Autodesk Fusion 360 part; units mm, degrees
(part 2 of 2)
sketch "Sketch4" plane through (0, 0, 6.35) normal (0, 0, 1) x (-1, 0, 0)
  circle A0 centre (2.4092, -3.6756) radius 2.1488
  arc A1 (-0.9894, -8.6855) -> (-1.1636, -11.2308) centre (2.9194, -10.2316) ccw
  arc A2 (-1.1636, -11.2308) -> (-0.826, -11.3814) centre (2.4092, -3.6756) ccw
  arc A3 (-0.826, -11.3814) -> (0.9516, -9.5514) centre (-2.8101, -7.6757) ccw
  spline S0 degree 5 poles (0.9516, -9.5514) (0.9679, -9.5486) (1.0003, -9.5432) (1.0488, -9.5361) (1.1133, -9.5282) (1.1934, -9.5212) (1.273, -9.5171) (1.3428, -9.5162) (1.3964, -9.5173) (1.4342, -9.5189) (1.4562, -9.5202) (1.4625, -9.5206) knots 0 0 0 0 0 0 0.066667 0.133333 0.2 0.266667 0.333333 0.4 0.426673 0.426673 0.426673 0.426673 0.426673 0.426673
  spline S1 degree 5 poles (1.4625, -9.5206) (1.472, -9.5212) (1.4971, -9.5229) (1.5284, -9.5254) (1.5597, -9.5286) (1.591, -9.5324) (1.6129, -9.5353) (1.6191, -9.5361) knots 0.426673 0.426673 0.426673 0.426673 0.426673 0.426673 0.466667 0.533333 0.559717 0.559717 0.559717 0.559717 0.559717 0.559717
  spline S2 degree 5 poles (1.6191, -9.5361) (1.6253, -9.537) (1.6472, -9.54) (1.6783, -9.5446) (1.7094, -9.5498) (1.7402, -9.5556) (1.7649, -9.5607) (1.7742, -9.5626) knots -0.559717 -0.559717 -0.559717 -0.559717 -0.559717 -0.559717 -0.533333 -0.466667 -0.426673 -0.426673 -0.426673 -0.426673 -0.426673 -0.426673
  spline S3 degree 5 poles (1.7742, -9.5626) (1.7804, -9.5639) (1.8019, -9.5685) (1.8388, -9.5769) (1.8908, -9.5901) (1.9578, -9.6094) (2.0336, -9.6344) (2.109, -9.6624) (2.169, -9.6871) (2.2139, -9.7068) (2.2438, -9.7206) (2.2587, -9.7276) knots -0.426673 -0.426673 -0.426673 -0.426673 -0.426673 -0.426673 -0.4 -0.333333 -0.266667 -0.2 -0.133333 -0.066667 0 0 0 0 0 0
  arc A4 (2.2587, -9.7276) -> (3.4882, -11.963) centre (6.3829, -8.915) ccw
  arc A5 (3.4882, -11.963) -> (3.8537, -11.9072) centre (2.4092, -3.6756) ccw
  arc A6 (3.8537, -11.9072) -> (4.3597, -9.4066) centre (0.181, -9.8625) ccw
  spline S4 degree 5 poles (4.3597, -9.4066) (4.3718, -9.3955) (4.3962, -9.3734) (4.4332, -9.3412) (4.4831, -9.2997) (4.5467, -9.2505) (4.6115, -9.204) (4.6697, -9.1656) (4.7154, -9.1375) (4.7481, -9.1184) (4.7673, -9.1076) (4.7728, -9.1045) knots 0 0 0 0 0 0 0.066667 0.133333 0.2 0.266667 0.333333 0.4 0.426673 0.426673 0.426673 0.426673 0.426673 0.426673
  spline S5 degree 5 poles (4.7728, -9.1045) (4.7811, -9.0999) (4.8031, -9.0877) (4.8309, -9.073) (4.8589, -9.0587) (4.8873, -9.045) (4.9073, -9.0356) (4.9129, -9.0329) knots 0.426673 0.426673 0.426673 0.426673 0.426673 0.426673 0.466667 0.533333 0.559717 0.559717 0.559717 0.559717 0.559717 0.559717
  spline S6 degree 5 poles (4.9129, -9.0329) (4.9186, -9.0303) (4.9386, -9.021) (4.9674, -9.008) (4.9963, -8.9957) (5.0254, -8.9838) (5.0489, -8.9747) (5.0577, -8.9714) knots -0.559717 -0.559717 -0.559717 -0.559717 -0.559717 -0.559717 -0.533333 -0.466667 -0.426673 -0.426673 -0.426673 -0.426673 -0.426673 -0.426673
  spline S7 degree 5 poles (5.0577, -8.9714) (5.0636, -8.9691) (5.0843, -8.9613) (5.1198, -8.9485) (5.1707, -8.9314) (5.2375, -8.9114) (5.3148, -8.8915) (5.3933, -8.8743) (5.4572, -8.8626) (5.5056, -8.855) (5.5382, -8.8504) (5.5545, -8.8482) knots -0.426673 -0.426673 -0.426673 -0.426673 -0.426673 -0.426673 -0.4 -0.333333 -0.266667 -0.2 -0.133333 -0.066667 0 0 0 0 0 0
  arc A7 (5.5545, -8.8482) -> (7.7974, -10.064) centre (8.5847, -5.9349) ccw
  arc A8 (7.7974, -10.064) -> (8.0747, -9.8195) centre (2.4092, -3.6756) ccw
  arc A9 (8.0747, -9.8195) -> (7.1484, -7.4423) centre (3.8796, -10.085) ccw
  spline S8 degree 5 poles (7.1484, -7.4423) (7.1526, -7.4263) (7.1613, -7.3946) (7.1749, -7.3475) (7.1945, -7.2856) (7.2214, -7.2098) (7.2508, -7.1357) (7.2789, -7.0719) (7.3022, -7.0235) (7.3194, -6.9899) (7.3297, -6.9704) (7.3327, -6.9648) knots 0 0 0 0 0 0 0.066667 0.133333 0.2 0.266667 0.333333 0.4 0.426673 0.426673 0.426673 0.426673 0.426673 0.426673
  spline S9 degree 5 poles (7.3327, -6.9648) (7.3371, -6.9564) (7.3491, -6.9343) (7.3645, -6.9069) (7.3804, -6.8797) (7.3968, -6.8528) (7.4085, -6.8341) (7.4119, -6.8288) knots 0.426673 0.426673 0.426673 0.426673 0.426673 0.426673 0.466667 0.533333 0.559717 0.559717 0.559717 0.559717 0.559717 0.559717
  spline S10 degree 5 poles (7.4119, -6.8288) (7.4152, -6.8235) (7.427, -6.8049) (7.4442, -6.7785) (7.4618, -6.7524) (7.4799, -6.7267) (7.4948, -6.7063) (7.5004, -6.6987) knots -0.559717 -0.559717 -0.559717 -0.559717 -0.559717 -0.559717 -0.533333 -0.466667 -0.426673 -0.426673 -0.426673 -0.426673 -0.426673 -0.426673
  spline S11 degree 5 poles (7.5004, -6.6987) (7.5041, -6.6937) (7.5173, -6.676) (7.5402, -6.6459) (7.5738, -6.604) (7.6192, -6.5511) (7.6735, -6.4926) (7.7302, -6.4357) (7.7776, -6.3913) (7.8142, -6.3587) (7.8391, -6.3372) (7.8517, -6.3266) knots -0.426673 -0.426673 -0.426673 -0.426673 -0.426673 -0.426673 -0.4 -0.333333 -0.266667 -0.2 -0.133333 -0.066667 0 0 0 0 0 0
  arc A10 (7.8517, -6.3266) -> (10.3959, -6.1368) centre (8.8258, -2.2375) ccw
  arc A11 (10.3959, -6.1368) -> (10.4969, -5.7811) centre (2.4092, -3.6756) ccw
  arc A12 (10.4969, -5.7811) -> (8.4325, -4.2821) centre (7.1113, -8.2725) ccw
  spline S12 degree 5 poles (8.4325, -4.2821) (8.4274, -4.2664) (8.4175, -4.2351) (8.4035, -4.188) (8.3866, -4.1254) (8.3682, -4.0471) (8.3529, -3.9688) (8.342, -3.9) (8.3355, -3.8467) (8.3318, -3.809) (8.3299, -3.7871) (8.3294, -3.7808) knots 0 0 0 0 0 0 0.066667 0.133333 0.2 0.266667 0.333333 0.4 0.426673 0.426673 0.426673 0.426673 0.426673 0.426673
  spline S13 degree 5 poles (8.3294, -3.7808) (8.3286, -3.7714) (8.3267, -3.7462) (8.3248, -3.7149) (8.3235, -3.6834) (8.3227, -3.6519) (8.3225, -3.6298) (8.3225, -3.6236) knots 0.426673 0.426673 0.426673 0.426673 0.426673 0.426673 0.466667 0.533333 0.559717 0.559717 0.559717 0.559717 0.559717 0.559717
  spline S14 degree 5 poles (8.3225, -3.6236) (8.3224, -3.6173) (8.3222, -3.5953) (8.3224, -3.5637) (8.3232, -3.5323) (8.3245, -3.5009) (8.326, -3.4757) (8.3266, -3.4663) knots -0.559717 -0.559717 -0.559717 -0.559717 -0.559717 -0.559717 -0.533333 -0.466667 -0.426673 -0.426673 -0.426673 -0.426673 -0.426673 -0.426673
  spline S15 degree 5 poles (8.3266, -3.4663) (8.327, -3.46) (8.3285, -3.438) (8.3316, -3.4003) (8.3372, -3.3469) (8.3468, -3.2779) (8.3608, -3.1993) (8.3777, -3.1207) (8.3936, -3.0578) (8.4068, -3.0105) (8.4161, -2.979) (8.4209, -2.9633) knots -0.426673 -0.426673 -0.426673 -0.426673 -0.426673 -0.426673 -0.4 -0.333333 -0.266667 -0.2 -0.133333 -0.066667 0 0 0 0 0 0
  arc A13 (8.4209, -2.9633) -> (10.4586, -1.4281) centre (7.0297, 1.0033) ccw
  arc A14 (10.4586, -1.4281) -> (10.3514, -1.0743) centre (2.4092, -3.6756) ccw
  arc A15 (10.3514, -1.0743) -> (7.8042, -0.9293) centre (8.8501, -5.0006) ccw
  spline S16 degree 5 poles (7.8042, -0.9293) (7.7915, -0.9189) (7.7662, -0.8979) (7.729, -0.8659) (7.6808, -0.8224) (7.6231, -0.7664) (7.5678, -0.7089) (7.5215, -0.6568) (7.4872, -0.6155) (7.4637, -0.5859) (7.4502, -0.5684) (7.4464, -0.5634) knots 0 0 0 0 0 0 0.066667 0.133333 0.2 0.266667 0.333333 0.4 0.426673 0.426673 0.426673 0.426673 0.426673 0.426673
  spline S17 degree 5 poles (7.4464, -0.5634) (7.4407, -0.5559) (7.4255, -0.5358) (7.4069, -0.5104) (7.3888, -0.4847) (7.3712, -0.4586) (7.359, -0.4401) (7.3556, -0.4349) knots 0.426673 0.426673 0.426673 0.426673 0.426673 0.426673 0.466667 0.533333 0.559717 0.559717 0.559717 0.559717 0.559717 0.559717
  spline S18 degree 5 poles (7.3556, -0.4349) (7.3522, -0.4296) (7.3401, -0.4112) (7.3232, -0.3846) (7.3069, -0.3577) (7.291, -0.3305) (7.2786, -0.3086) (7.2741, -0.3003) knots -0.559717 -0.559717 -0.559717 -0.559717 -0.559717 -0.559717 -0.533333 -0.466667 -0.426673 -0.426673 -0.426673 -0.426673 -0.426673 -0.426673
  spline S19 degree 5 poles (7.2741, -0.3003) (7.271, -0.2948) (7.2604, -0.2755) (7.2426, -0.2421) (7.2184, -0.1942) (7.1892, -0.1309) (7.1585, -0.0573) (7.1302, 0.018) (7.1096, 0.0796) (7.0951, 0.1264) (7.0859, 0.158) (7.0814, 0.1739) knots -0.426673 -0.426673 -0.426673 -0.426673 -0.426673 -0.426673 -0.4 -0.333333 -0.266667 -0.2 -0.133333 -0.066667 0 0 0 0 0 0
  arc A16 (7.0814, 0.1739) -> (7.9657, 2.567) centre (3.7666, 2.7586) ccw
  arc A17 (7.9657, 2.567) -> (7.6842, 2.8066) centre (2.4092, -3.6756) ccw
  arc A18 (7.6842, 2.8066) -> (5.463, 1.5515) centre (8.544, -1.308) ccw
  spline S20 degree 5 poles (5.463, 1.5515) (5.4466, 1.5534) (5.414, 1.5574) (5.3654, 1.5642) (5.3014, 1.5748) (5.2226, 1.5906) (5.145, 1.6092) (5.0778, 1.6279) (5.0267, 1.6441) (4.9909, 1.6563) (4.9701, 1.6638) (4.9642, 1.6659) knots 0 0 0 0 0 0 0.066667 0.133333 0.2 0.266667 0.333333 0.4 0.426673 0.426673 0.426673 0.426673 0.426673 0.426673
  spline S21 degree 5 poles (4.9642, 1.6659) (4.9553, 1.6691) (4.9316, 1.6778) (4.9023, 1.6891) (4.8732, 1.701) (4.8442, 1.7134) (4.824, 1.7224) (4.8183, 1.7249) knots 0.426673 0.426673 0.426673 0.426673 0.426673 0.426673 0.466667 0.533333 0.559717 0.559717 0.559717 0.559717 0.559717 0.559717
  spline S22 degree 5 poles (4.8183, 1.7249) (4.8126, 1.7275) (4.7924, 1.7365) (4.7639, 1.7498) (4.7356, 1.7635) (4.7076, 1.7778) (4.6853, 1.7896) (4.677, 1.794) knots -0.559717 -0.559717 -0.559717 -0.559717 -0.559717 -0.559717 -0.533333 -0.466667 -0.426673 -0.426673 -0.426673 -0.426673 -0.426673 -0.426673
  spline S23 degree 5 poles (4.677, 1.794) (4.6714, 1.797) (4.652, 1.8075) (4.619, 1.826) (4.5728, 1.8533) (4.5139, 1.8907) (4.4483, 1.936) (4.3839, 1.9841) (4.3332, 2.0247) (4.2957, 2.0563) (4.2709, 2.0779) (4.2586, 2.0888) knots -0.426673 -0.426673 -0.426673 -0.426673 -0.426673 -0.426673 -0.4 -0.333333 -0.266667 -0.2 -0.133333 -0.066667 0 0 0 0 0 0
  arc A19 (4.2586, 2.0888) -> (3.7086, 4.5801) centre (0.0725, 2.4711) ccw
  arc A20 (3.7086, 4.5801) -> (3.3423, 4.6295) centre (2.4092, -3.6756) ccw
  arc A21 (3.3423, 4.6295) -> (2.1522, 2.3728) centre (6.2901, 1.6329) ccw
  spline S24 degree 5 poles (2.1522, 2.3728) (2.1374, 2.3655) (2.1078, 2.3512) (2.0633, 2.3307) (2.0037, 2.305) (1.9288, 2.2757) (1.8535, 2.2493) (1.7869, 2.2288) (1.7351, 2.2148) (1.6983, 2.2057) (1.6769, 2.2007) (1.6707, 2.1993) knots 0 0 0 0 0 0 0.066667 0.133333 0.2 0.266667 0.333333 0.4 0.426673 0.426673 0.426673 0.426673 0.426673 0.426673
  spline S25 degree 5 poles (1.6707, 2.1993) (1.6615, 2.1972) (1.6369, 2.1917) (1.6061, 2.1854) (1.5752, 2.1796) (1.5441, 2.1744) (1.5223, 2.171) (1.5161, 2.1701) knots 0.426673 0.426673 0.426673 0.426673 0.426673 0.426673 0.466667 0.533333 0.559717 0.559717 0.559717 0.559717 0.559717 0.559717
  spline S26 degree 5 poles (1.5161, 2.1701) (1.5099, 2.1691) (1.4881, 2.1659) (1.4569, 2.1616) (1.4256, 2.1578) (1.3944, 2.1547) (1.3693, 2.1526) (1.3598, 2.1518) knots -0.559717 -0.559717 -0.559717 -0.559717 -0.559717 -0.559717 -0.533333 -0.466667 -0.426673 -0.426673 -0.426673 -0.426673 -0.426673 -0.426673
  spline S27 degree 5 poles (1.3598, 2.1518) (1.3536, 2.1513) (1.3316, 2.1497) (1.2938, 2.1473) (1.2402, 2.1453) (1.1704, 2.145) (1.0907, 2.1476) (1.0105, 2.1532) (0.9459, 2.16) (0.8973, 2.1663) (0.8648, 2.1711) (0.8485, 2.1736) knots -0.426673 -0.426673 -0.426673 -0.426673 -0.426673 -0.426673 -0.4 -0.333333 -0.266667 -0.2 -0.133333 -0.066667 0 0 0 0 0 0
  arc A22 (0.8485, 2.1736) -> (-0.961, 3.9721) centre (-2.8797, 0.232) ccw
  arc A23 (-0.961, 3.9721) -> (-1.2959, 3.8155) centre (2.4092, -3.6756) ccw
  arc A24 (-1.2959, 3.8155) -> (-1.077, 1.2737) centre (2.804, 2.8884) ccw
  spline S28 degree 5 poles (-1.077, 1.2737) (-1.0855, 1.2596) (-1.1027, 1.2316) (-1.1291, 1.1902) (-1.1653, 1.1364) (-1.2125, 1.0712) (-1.2615, 1.0084) (-1.3065, 0.9551) (-1.3425, 0.9152) (-1.3685, 0.8878) (-1.3839, 0.872) (-1.3883, 0.8675) knots 0 0 0 0 0 0 0.066667 0.133333 0.2 0.266667 0.333333 0.4 0.426673 0.426673 0.426673 0.426673 0.426673 0.426673
  spline S29 degree 5 poles (-1.3883, 0.8675) (-1.3949, 0.8607) (-1.4126, 0.8428) (-1.4351, 0.8208) (-1.458, 0.7993) (-1.4813, 0.7781) (-1.4979, 0.7634) (-1.5026, 0.7593) knots 0.426673 0.426673 0.426673 0.426673 0.426673 0.426673 0.466667 0.533333 0.559717 0.559717 0.559717 0.559717 0.559717 0.559717
  spline S30 degree 5 poles (-1.5026, 0.7593) (-1.5072, 0.7552) (-1.5238, 0.7406) (-1.5478, 0.7201) (-1.572, 0.7001) (-1.5966, 0.6805) (-1.6166, 0.6651) (-1.6241, 0.6594) knots -0.559717 -0.559717 -0.559717 -0.559717 -0.559717 -0.559717 -0.533333 -0.466667 -0.426673 -0.426673 -0.426673 -0.426673 -0.426673 -0.426673
  spline S31 degree 5 poles (-1.6241, 0.6594) (-1.6291, 0.6556) (-1.6468, 0.6423) (-1.6773, 0.62) (-1.7213, 0.5893) (-1.7798, 0.5513) (-1.8483, 0.5104) (-1.9188, 0.4718) (-1.9767, 0.4425) (-2.0211, 0.4216) (-2.051, 0.408) (-2.0661, 0.4013) knots -0.426673 -0.426673 -0.426673 -0.426673 -0.426673 -0.426673 -0.4 -0.333333 -0.266667 -0.2 -0.133333 -0.066667 0 0 0 0 0 0
  arc A25 (-2.0661, 0.4013) -> (-4.5607, 0.936) centre (-4.1528, -3.2477) ccw
  arc A26 (-4.5607, 0.936) -> (-4.7578, 0.6232) centre (2.4092, -3.6756) ccw
  arc A27 (-4.7578, 0.6232) -> (-3.1994, -1.3967) centre (-0.8075, 2.0598) ccw
  spline S32 degree 5 poles (-3.1994, -1.3967) (-3.1989, -1.4132) (-3.1982, -1.4461) (-3.1981, -1.4951) (-3.1994, -1.56) (-3.2039, -1.6403) (-3.2112, -1.7197) (-3.2202, -1.7889) (-3.2289, -1.8418) (-3.2359, -1.879) (-3.2403, -1.9006) (-3.2416, -1.9068) knots 0 0 0 0 0 0 0.066667 0.133333 0.2 0.266667 0.333333 0.4 0.426673 0.426673 0.426673 0.426673 0.426673 0.426673
  spline S33 degree 5 poles (-3.2416, -1.9068) (-3.2435, -1.916) (-3.2488, -1.9407) (-3.2558, -1.9713) (-3.2634, -2.0019) (-3.2716, -2.0323) (-3.2776, -2.0535) (-3.2793, -2.0596) knots 0.426673 0.426673 0.426673 0.426673 0.426673 0.426673 0.466667 0.533333 0.559717 0.559717 0.559717 0.559717 0.559717 0.559717
  spline S34 degree 5 poles (-3.2793, -2.0596) (-3.281, -2.0656) (-3.2871, -2.0868) (-3.2961, -2.117) (-3.3057, -2.1469) (-3.3158, -2.1767) (-3.3243, -2.2004) (-3.3276, -2.2093) knots -0.559717 -0.559717 -0.559717 -0.559717 -0.559717 -0.559717 -0.533333 -0.466667 -0.426673 -0.426673 -0.426673 -0.426673 -0.426673 -0.426673
  spline S35 degree 5 poles (-3.3276, -2.2093) (-3.3297, -2.2152) (-3.3373, -2.2359) (-3.3509, -2.2712) (-3.3713, -2.3209) (-3.4, -2.3844) (-3.4356, -2.4558) (-3.474, -2.5265) (-3.5069, -2.5824) (-3.5329, -2.624) (-3.5507, -2.6516) (-3.5598, -2.6654) knots -0.426673 -0.426673 -0.426673 -0.426673 -0.426673 -0.426673 -0.4 -0.333333 -0.266667 -0.2 -0.133333 -0.066667 0 0 0 0 0 0
  arc A28 (-3.5598, -2.6654) -> (-5.9474, -3.5643) centre (-3.3425, -6.8632) ccw
  arc A29 (-5.9474, -3.5643) -> (-5.9442, -3.9339) centre (2.4092, -3.6756) ccw
  arc A30 (-5.9442, -3.9339) -> (-3.5411, -4.7907) centre (-3.3976, -0.5897) ccw
  spline S36 degree 5 poles (-3.5411, -4.7907) (-3.5318, -4.8043) (-3.5135, -4.8316) (-3.4868, -4.8727) (-3.4528, -4.9281) (-3.4132, -4.998) (-3.3764, -5.0688) (-3.3466, -5.1318) (-3.3253, -5.1811) (-3.3111, -5.2162) (-3.3031, -5.2367) (-3.3009, -5.2426) knots 0 0 0 0 0 0 0.066667 0.133333 0.2 0.266667 0.333333 0.4 0.426673 0.426673 0.426673 0.426673 0.426673 0.426673
  spline S37 degree 5 poles (-3.3009, -5.2426) (-3.2975, -5.2514) (-3.2886, -5.275) (-3.2779, -5.3046) (-3.2678, -5.3344) (-3.2582, -5.3644) (-3.2518, -5.3855) (-3.25, -5.3915) knots 0.426673 0.426673 0.426673 0.426673 0.426673 0.426673 0.466667 0.533333 0.559717 0.559717 0.559717 0.559717 0.559717 0.559717
  spline S38 degree 5 poles (-3.25, -5.3915) (-3.2481, -5.3975) (-3.2418, -5.4186) (-3.2331, -5.4489) (-3.2249, -5.4793) (-3.2174, -5.5098) (-3.2117, -5.5344) (-3.2096, -5.5436) knots -0.559717 -0.559717 -0.559717 -0.559717 -0.559717 -0.559717 -0.533333 -0.466667 -0.426673 -0.426673 -0.426673 -0.426673 -0.426673 -0.426673
  spline S39 degree 5 poles (-3.2096, -5.5436) (-3.2082, -5.5497) (-3.2035, -5.5713) (-3.1958, -5.6083) (-3.1861, -5.6611) (-3.1759, -5.7301) (-3.1672, -5.8094) (-3.1613, -5.8895) (-3.1588, -5.9544) (-3.1581, -6.0035) (-3.1582, -6.0363) (-3.1584, -6.0528) knots -0.426673 -0.426673 -0.426673 -0.426673 -0.426673 -0.426673 -0.4 -0.333333 -0.266667 -0.2 -0.133333 -0.066667 0 0 0 0 0 0
  arc A31 (-3.1584, -6.0528) -> (-4.6811, -8.0999) centre (-0.706, -9.4668) ccw
  arc A32 (-4.6811, -8.0999) -> (-4.4785, -8.4091) centre (2.4092, -3.6756) ccw
  arc A33 (-4.4785, -8.4091) -> (-1.9937, -7.8306) centre (-4.1442, -4.2189) ccw
  spline S40 degree 5 poles (-1.9937, -7.8306) (-1.9785, -7.837) (-1.9483, -7.8501) (-1.9036, -7.8703) (-1.8451, -7.8985) (-1.774, -7.9359) (-1.7048, -7.9755) (-1.6456, -8.0125) (-1.6011, -8.0424) (-1.5702, -8.0642) (-1.5523, -8.0772) (-1.5472, -8.0809) knots 0 0 0 0 0 0 0.066667 0.133333 0.2 0.266667 0.333333 0.4 0.426673 0.426673 0.426673 0.426673 0.426673 0.426673
  spline S41 degree 5 poles (-1.5472, -8.0809) (-1.5396, -8.0865) (-1.5194, -8.1015) (-1.4944, -8.1206) (-1.4698, -8.1402) (-1.4455, -8.1603) (-1.4287, -8.1746) (-1.4239, -8.1787) knots 0.426673 0.426673 0.426673 0.426673 0.426673 0.426673 0.466667 0.533333 0.559717 0.559717 0.559717 0.559717 0.559717 0.559717
  spline S42 degree 5 poles (-1.4239, -8.1787) (-1.4192, -8.1827) (-1.4024, -8.197) (-1.3787, -8.2178) (-1.3554, -8.239) (-1.3325, -8.2606) (-1.3145, -8.2781) (-1.3078, -8.2848) knots -0.559717 -0.559717 -0.559717 -0.559717 -0.559717 -0.559717 -0.533333 -0.466667 -0.426673 -0.426673 -0.426673 -0.426673 -0.426673 -0.426673
  spline S43 degree 5 poles (-1.3078, -8.2848) (-1.3033, -8.2892) (-1.2876, -8.3047) (-1.2611, -8.3318) (-1.2245, -8.371) (-1.1786, -8.4234) (-1.1284, -8.4854) (-1.0801, -8.5497) (-1.0429, -8.6029) (-1.0158, -8.6438) (-0.9981, -8.6715) (-0.9894, -8.6855) knots -0.426673 -0.426673 -0.426673 -0.426673 -0.426673 -0.426673 -0.4 -0.333333 -0.266667 -0.2 -0.133333 -0.066667 0 0 0 0 0 0
  circle A34 centre (2.4092, -3.6756) radius 2.3876
  dimension "d9" = 4.7752
  constraint concentric A0 A34
  measures "d9" diameter of A34
extrude "Extrude3" cut sketch "Sketch4" against normal blind 12.7 contours A34
sketch "Sketch5" plane through (0, 0, 6.35) normal (0, 0, 1) x (-1, 0, 0)
  circle A0 centre (2.4092, -3.6756) radius 2.3876
  arc A1 (-0.9894, -8.6855) -> (-1.1636, -11.2308) centre (2.9194, -10.2316) ccw
  arc A2 (-1.1636, -11.2308) -> (-0.826, -11.3814) centre (2.4092, -3.6756) ccw
  arc A3 (-0.826, -11.3814) -> (0.9516, -9.5514) centre (-2.8101, -7.6757) ccw
  spline S0 degree 5 poles (0.9516, -9.5514) (0.9679, -9.5486) (1.0003, -9.5432) (1.0488, -9.5361) (1.1133, -9.5282) (1.1934, -9.5212) (1.273, -9.5171) (1.3428, -9.5162) (1.3964, -9.5173) (1.4342, -9.5189) (1.4562, -9.5202) (1.4625, -9.5206) knots 0 0 0 0 0 0 0.066667 0.133333 0.2 0.266667 0.333333 0.4 0.426673 0.426673 0.426673 0.426673 0.426673 0.426673
  spline S1 degree 5 poles (1.4625, -9.5206) (1.472, -9.5212) (1.4971, -9.5229) (1.5284, -9.5254) (1.5597, -9.5286) (1.591, -9.5324) (1.6129, -9.5353) (1.6191, -9.5361) knots 0.426673 0.426673 0.426673 0.426673 0.426673 0.426673 0.466667 0.533333 0.559717 0.559717 0.559717 0.559717 0.559717 0.559717
  spline S2 degree 5 poles (1.6191, -9.5361) (1.6253, -9.537) (1.6472, -9.54) (1.6783, -9.5446) (1.7094, -9.5498) (1.7402, -9.5556) (1.7649, -9.5607) (1.7742, -9.5626) knots -0.559717 -0.559717 -0.559717 -0.559717 -0.559717 -0.559717 -0.533333 -0.466667 -0.426673 -0.426673 -0.426673 -0.426673 -0.426673 -0.426673
  spline S3 degree 5 poles (1.7742, -9.5626) (1.7804, -9.5639) (1.8019, -9.5685) (1.8388, -9.5769) (1.8908, -9.5901) (1.9578, -9.6094) (2.0336, -9.6344) (2.109, -9.6624) (2.169, -9.6871) (2.2139, -9.7068) (2.2438, -9.7206) (2.2587, -9.7276) knots -0.426673 -0.426673 -0.426673 -0.426673 -0.426673 -0.426673 -0.4 -0.333333 -0.266667 -0.2 -0.133333 -0.066667 0 0 0 0 0 0
  arc A4 (2.2587, -9.7276) -> (3.4882, -11.963) centre (6.3829, -8.915) ccw
  arc A5 (3.4882, -11.963) -> (3.8537, -11.9072) centre (2.4092, -3.6756) ccw
  arc A6 (3.8537, -11.9072) -> (4.3597, -9.4066) centre (0.181, -9.8625) ccw
  spline S4 degree 5 poles (4.3597, -9.4066) (4.3718, -9.3955) (4.3962, -9.3734) (4.4332, -9.3412) (4.4831, -9.2997) (4.5467, -9.2505) (4.6115, -9.204) (4.6697, -9.1656) (4.7154, -9.1375) (4.7481, -9.1184) (4.7673, -9.1076) (4.7728, -9.1045) knots 0 0 0 0 0 0 0.066667 0.133333 0.2 0.266667 0.333333 0.4 0.426673 0.426673 0.426673 0.426673 0.426673 0.426673
  spline S5 degree 5 poles (4.7728, -9.1045) (4.7811, -9.0999) (4.8031, -9.0877) (4.8309, -9.073) (4.8589, -9.0587) (4.8873, -9.045) (4.9073, -9.0356) (4.9129, -9.0329) knots 0.426673 0.426673 0.426673 0.426673 0.426673 0.426673 0.466667 0.533333 0.559717 0.559717 0.559717 0.559717 0.559717 0.559717
  spline S6 degree 5 poles (4.9129, -9.0329) (4.9186, -9.0303) (4.9386, -9.021) (4.9674, -9.008) (4.9963, -8.9957) (5.0254, -8.9838) (5.0489, -8.9747) (5.0577, -8.9714) knots -0.559717 -0.559717 -0.559717 -0.559717 -0.559717 -0.559717 -0.533333 -0.466667 -0.426673 -0.426673 -0.426673 -0.426673 -0.426673 -0.426673
  spline S7 degree 5 poles (5.0577, -8.9714) (5.0636, -8.9691) (5.0843, -8.9613) (5.1198, -8.9485) (5.1707, -8.9314) (5.2375, -8.9114) (5.3148, -8.8915) (5.3933, -8.8743) (5.4572, -8.8626) (5.5056, -8.855) (5.5382, -8.8504) (5.5545, -8.8482) knots -0.426673 -0.426673 -0.426673 -0.426673 -0.426673 -0.426673 -0.4 -0.333333 -0.266667 -0.2 -0.133333 -0.066667 0 0 0 0 0 0
  arc A7 (5.5545, -8.8482) -> (7.7974, -10.064) centre (8.5847, -5.9349) ccw
  arc A8 (7.7974, -10.064) -> (8.0747, -9.8195) centre (2.4092, -3.6756) ccw
  arc A9 (8.0747, -9.8195) -> (7.1484, -7.4423) centre (3.8796, -10.085) ccw
  spline S8 degree 5 poles (7.1484, -7.4423) (7.1526, -7.4263) (7.1613, -7.3946) (7.1749, -7.3475) (7.1945, -7.2856) (7.2214, -7.2098) (7.2508, -7.1357) (7.2789, -7.0719) (7.3022, -7.0235) (7.3194, -6.9899) (7.3297, -6.9704) (7.3327, -6.9648) knots 0 0 0 0 0 0 0.066667 0.133333 0.2 0.266667 0.333333 0.4 0.426673 0.426673 0.426673 0.426673 0.426673 0.426673
  spline S9 degree 5 poles (7.3327, -6.9648) (7.3371, -6.9564) (7.3491, -6.9343) (7.3645, -6.9069) (7.3804, -6.8797) (7.3968, -6.8528) (7.4085, -6.8341) (7.4119, -6.8288) knots 0.426673 0.426673 0.426673 0.426673 0.426673 0.426673 0.466667 0.533333 0.559717 0.559717 0.559717 0.559717 0.559717 0.559717
  spline S10 degree 5 poles (7.4119, -6.8288) (7.4152, -6.8235) (7.427, -6.8049) (7.4442, -6.7785) (7.4618, -6.7524) (7.4799, -6.7267) (7.4948, -6.7063) (7.5004, -6.6987) knots -0.559717 -0.559717 -0.559717 -0.559717 -0.559717 -0.559717 -0.533333 -0.466667 -0.426673 -0.426673 -0.426673 -0.426673 -0.426673 -0.426673
  spline S11 degree 5 poles (7.5004, -6.6987) (7.5041, -6.6937) (7.5173, -6.676) (7.5402, -6.6459) (7.5738, -6.604) (7.6192, -6.5511) (7.6735, -6.4926) (7.7302, -6.4357) (7.7776, -6.3913) (7.8142, -6.3587) (7.8391, -6.3372) (7.8517, -6.3266) knots -0.426673 -0.426673 -0.426673 -0.426673 -0.426673 -0.426673 -0.4 -0.333333 -0.266667 -0.2 -0.133333 -0.066667 0 0 0 0 0 0
  arc A10 (7.8517, -6.3266) -> (10.3959, -6.1368) centre (8.8258, -2.2375) ccw
  arc A11 (10.3959, -6.1368) -> (10.4969, -5.7811) centre (2.4092, -3.6756) ccw
  arc A12 (10.4969, -5.7811) -> (8.4325, -4.2821) centre (7.1113, -8.2725) ccw
  spline S12 degree 5 poles (8.4325, -4.2821) (8.4274, -4.2664) (8.4175, -4.2351) (8.4035, -4.188) (8.3866, -4.1254) (8.3682, -4.0471) (8.3529, -3.9688) (8.342, -3.9) (8.3355, -3.8467) (8.3318, -3.809) (8.3299, -3.7871) (8.3294, -3.7808) knots 0 0 0 0 0 0 0.066667 0.133333 0.2 0.266667 0.333333 0.4 0.426673 0.426673 0.426673 0.426673 0.426673 0.426673
  spline S13 degree 5 poles (8.3294, -3.7808) (8.3286, -3.7714) (8.3267, -3.7462) (8.3248, -3.7149) (8.3235, -3.6834) (8.3227, -3.6519) (8.3225, -3.6298) (8.3225, -3.6236) knots 0.426673 0.426673 0.426673 0.426673 0.426673 0.426673 0.466667 0.533333 0.559717 0.559717 0.559717 0.559717 0.559717 0.559717
  spline S14 degree 5 poles (8.3225, -3.6236) (8.3224, -3.6173) (8.3222, -3.5953) (8.3224, -3.5637) (8.3232, -3.5323) (8.3245, -3.5009) (8.326, -3.4757) (8.3266, -3.4663) knots -0.559717 -0.559717 -0.559717 -0.559717 -0.559717 -0.559717 -0.533333 -0.466667 -0.426673 -0.426673 -0.426673 -0.426673 -0.426673 -0.426673
  spline S15 degree 5 poles (8.3266, -3.4663) (8.327, -3.46) (8.3285, -3.438) (8.3316, -3.4003) (8.3372, -3.3469) (8.3468, -3.2779) (8.3608, -3.1993) (8.3777, -3.1207) (8.3936, -3.0578) (8.4068, -3.0105) (8.4161, -2.979) (8.4209, -2.9633) knots -0.426673 -0.426673 -0.426673 -0.426673 -0.426673 -0.426673 -0.4 -0.333333 -0.266667 -0.2 -0.133333 -0.066667 0 0 0 0 0 0
  arc A13 (8.4209, -2.9633) -> (10.4586, -1.4281) centre (7.0297, 1.0033) ccw
  arc A14 (10.4586, -1.4281) -> (10.3514, -1.0743) centre (2.4092, -3.6756) ccw
  arc A15 (10.3514, -1.0743) -> (7.8042, -0.9293) centre (8.8501, -5.0006) ccw
  spline S16 degree 5 poles (7.8042, -0.9293) (7.7915, -0.9189) (7.7662, -0.8979) (7.729, -0.8659) (7.6808, -0.8224) (7.6231, -0.7664) (7.5678, -0.7089) (7.5215, -0.6568) (7.4872, -0.6155) (7.4637, -0.5859) (7.4502, -0.5684) (7.4464, -0.5634) knots 0 0 0 0 0 0 0.066667 0.133333 0.2 0.266667 0.333333 0.4 0.426673 0.426673 0.426673 0.426673 0.426673 0.426673
  spline S17 degree 5 poles (7.4464, -0.5634) (7.4407, -0.5559) (7.4255, -0.5358) (7.4069, -0.5104) (7.3888, -0.4847) (7.3712, -0.4586) (7.359, -0.4401) (7.3556, -0.4349) knots 0.426673 0.426673 0.426673 0.426673 0.426673 0.426673 0.466667 0.533333 0.559717 0.559717 0.559717 0.559717 0.559717 0.559717
  spline S18 degree 5 poles (7.3556, -0.4349) (7.3522, -0.4296) (7.3401, -0.4112) (7.3232, -0.3846) (7.3069, -0.3577) (7.291, -0.3305) (7.2786, -0.3086) (7.2741, -0.3003) knots -0.559717 -0.559717 -0.559717 -0.559717 -0.559717 -0.559717 -0.533333 -0.466667 -0.426673 -0.426673 -0.426673 -0.426673 -0.426673 -0.426673
  spline S19 degree 5 poles (7.2741, -0.3003) (7.271, -0.2948) (7.2604, -0.2755) (7.2426, -0.2421) (7.2184, -0.1942) (7.1892, -0.1309) (7.1585, -0.0573) (7.1302, 0.018) (7.1096, 0.0796) (7.0951, 0.1264) (7.0859, 0.158) (7.0814, 0.1739) knots -0.426673 -0.426673 -0.426673 -0.426673 -0.426673 -0.426673 -0.4 -0.333333 -0.266667 -0.2 -0.133333 -0.066667 0 0 0 0 0 0
  arc A16 (7.0814, 0.1739) -> (7.9657, 2.567) centre (3.7666, 2.7586) ccw
  arc A17 (7.9657, 2.567) -> (7.6842, 2.8066) centre (2.4092, -3.6756) ccw
  arc A18 (7.6842, 2.8066) -> (5.463, 1.5515) centre (8.544, -1.308) ccw
  spline S20 degree 5 poles (5.463, 1.5515) (5.4466, 1.5534) (5.414, 1.5574) (5.3654, 1.5642) (5.3014, 1.5748) (5.2226, 1.5906) (5.145, 1.6092) (5.0778, 1.6279) (5.0267, 1.6441) (4.9909, 1.6563) (4.9701, 1.6638) (4.9642, 1.6659) knots 0 0 0 0 0 0 0.066667 0.133333 0.2 0.266667 0.333333 0.4 0.426673 0.426673 0.426673 0.426673 0.426673 0.426673
  spline S21 degree 5 poles (4.9642, 1.6659) (4.9553, 1.6691) (4.9316, 1.6778) (4.9023, 1.6891) (4.8732, 1.701) (4.8442, 1.7134) (4.824, 1.7224) (4.8183, 1.7249) knots 0.426673 0.426673 0.426673 0.426673 0.426673 0.426673 0.466667 0.533333 0.559717 0.559717 0.559717 0.559717 0.559717 0.559717
  spline S22 degree 5 poles (4.8183, 1.7249) (4.8126, 1.7275) (4.7924, 1.7365) (4.7639, 1.7498) (4.7356, 1.7635) (4.7076, 1.7778) (4.6853, 1.7896) (4.677, 1.794) knots -0.559717 -0.559717 -0.559717 -0.559717 -0.559717 -0.559717 -0.533333 -0.466667 -0.426673 -0.426673 -0.426673 -0.426673 -0.426673 -0.426673
  spline S23 degree 5 poles (4.677, 1.794) (4.6714, 1.797) (4.652, 1.8075) (4.619, 1.826) (4.5728, 1.8533) (4.5139, 1.8907) (4.4483, 1.936) (4.3839, 1.9841) (4.3332, 2.0247) (4.2957, 2.0563) (4.2709, 2.0779) (4.2586, 2.0888) knots -0.426673 -0.426673 -0.426673 -0.426673 -0.426673 -0.426673 -0.4 -0.333333 -0.266667 -0.2 -0.133333 -0.066667 0 0 0 0 0 0
  arc A19 (4.2586, 2.0888) -> (3.7086, 4.5801) centre (0.0725, 2.4711) ccw
  arc A20 (3.7086, 4.5801) -> (3.3423, 4.6295) centre (2.4092, -3.6756) ccw
  arc A21 (3.3423, 4.6295) -> (2.1522, 2.3728) centre (6.2901, 1.6329) ccw
  spline S24 degree 5 poles (2.1522, 2.3728) (2.1374, 2.3655) (2.1078, 2.3512) (2.0633, 2.3307) (2.0037, 2.305) (1.9288, 2.2757) (1.8535, 2.2493) (1.7869, 2.2288) (1.7351, 2.2148) (1.6983, 2.2057) (1.6769, 2.2007) (1.6707, 2.1993) knots 0 0 0 0 0 0 0.066667 0.133333 0.2 0.266667 0.333333 0.4 0.426673 0.426673 0.426673 0.426673 0.426673 0.426673
  spline S25 degree 5 poles (1.6707, 2.1993) (1.6615, 2.1972) (1.6369, 2.1917) (1.6061, 2.1854) (1.5752, 2.1796) (1.5441, 2.1744) (1.5223, 2.171) (1.5161, 2.1701) knots 0.426673 0.426673 0.426673 0.426673 0.426673 0.426673 0.466667 0.533333 0.559717 0.559717 0.559717 0.559717 0.559717 0.559717
  spline S26 degree 5 poles (1.5161, 2.1701) (1.5099, 2.1691) (1.4881, 2.1659) (1.4569, 2.1616) (1.4256, 2.1578) (1.3944, 2.1547) (1.3693, 2.1526) (1.3598, 2.1518) knots -0.559717 -0.559717 -0.559717 -0.559717 -0.559717 -0.559717 -0.533333 -0.466667 -0.426673 -0.426673 -0.426673 -0.426673 -0.426673 -0.426673
  spline S27 degree 5 poles (1.3598, 2.1518) (1.3536, 2.1513) (1.3316, 2.1497) (1.2938, 2.1473) (1.2402, 2.1453) (1.1704, 2.145) (1.0907, 2.1476) (1.0105, 2.1532) (0.9459, 2.16) (0.8973, 2.1663) (0.8648, 2.1711) (0.8485, 2.1736) knots -0.426673 -0.426673 -0.426673 -0.426673 -0.426673 -0.426673 -0.4 -0.333333 -0.266667 -0.2 -0.133333 -0.066667 0 0 0 0 0 0
  arc A22 (0.8485, 2.1736) -> (-0.961, 3.9721) centre (-2.8797, 0.232) ccw
  arc A23 (-0.961, 3.9721) -> (-1.2959, 3.8155) centre (2.4092, -3.6756) ccw
  arc A24 (-1.2959, 3.8155) -> (-1.077, 1.2737) centre (2.804, 2.8884) ccw
  spline S28 degree 5 poles (-1.077, 1.2737) (-1.0855, 1.2596) (-1.1027, 1.2316) (-1.1291, 1.1902) (-1.1653, 1.1364) (-1.2125, 1.0712) (-1.2615, 1.0084) (-1.3065, 0.9551) (-1.3425, 0.9152) (-1.3685, 0.8878) (-1.3839, 0.872) (-1.3883, 0.8675) knots 0 0 0 0 0 0 0.066667 0.133333 0.2 0.266667 0.333333 0.4 0.426673 0.426673 0.426673 0.426673 0.426673 0.426673
  spline S29 degree 5 poles (-1.3883, 0.8675) (-1.3949, 0.8607) (-1.4126, 0.8428) (-1.4351, 0.8208) (-1.458, 0.7993) (-1.4813, 0.7781) (-1.4979, 0.7634) (-1.5026, 0.7593) knots 0.426673 0.426673 0.426673 0.426673 0.426673 0.426673 0.466667 0.533333 0.559717 0.559717 0.559717 0.559717 0.559717 0.559717
  spline S30 degree 5 poles (-1.5026, 0.7593) (-1.5072, 0.7552) (-1.5238, 0.7406) (-1.5478, 0.7201) (-1.572, 0.7001) (-1.5966, 0.6805) (-1.6166, 0.6651) (-1.6241, 0.6594) knots -0.559717 -0.559717 -0.559717 -0.559717 -0.559717 -0.559717 -0.533333 -0.466667 -0.426673 -0.426673 -0.426673 -0.426673 -0.426673 -0.426673
  spline S31 degree 5 poles (-1.6241, 0.6594) (-1.6291, 0.6556) (-1.6468, 0.6423) (-1.6773, 0.62) (-1.7213, 0.5893) (-1.7798, 0.5513) (-1.8483, 0.5104) (-1.9188, 0.4718) (-1.9767, 0.4425) (-2.0211, 0.4216) (-2.051, 0.408) (-2.0661, 0.4013) knots -0.426673 -0.426673 -0.426673 -0.426673 -0.426673 -0.426673 -0.4 -0.333333 -0.266667 -0.2 -0.133333 -0.066667 0 0 0 0 0 0
  arc A25 (-2.0661, 0.4013) -> (-4.5607, 0.936) centre (-4.1528, -3.2477) ccw
  arc A26 (-4.5607, 0.936) -> (-4.7578, 0.6232) centre (2.4092, -3.6756) ccw
  arc A27 (-4.7578, 0.6232) -> (-3.1994, -1.3967) centre (-0.8075, 2.0598) ccw
  spline S32 degree 5 poles (-3.1994, -1.3967) (-3.1989, -1.4132) (-3.1982, -1.4461) (-3.1981, -1.4951) (-3.1994, -1.56) (-3.2039, -1.6403) (-3.2112, -1.7197) (-3.2202, -1.7889) (-3.2289, -1.8418) (-3.2359, -1.879) (-3.2403, -1.9006) (-3.2416, -1.9068) knots 0 0 0 0 0 0 0.066667 0.133333 0.2 0.266667 0.333333 0.4 0.426673 0.426673 0.426673 0.426673 0.426673 0.426673
  spline S33 degree 5 poles (-3.2416, -1.9068) (-3.2435, -1.916) (-3.2488, -1.9407) (-3.2558, -1.9713) (-3.2634, -2.0019) (-3.2716, -2.0323) (-3.2776, -2.0535) (-3.2793, -2.0596) knots 0.426673 0.426673 0.426673 0.426673 0.426673 0.426673 0.466667 0.533333 0.559717 0.559717 0.559717 0.559717 0.559717 0.559717
  spline S34 degree 5 poles (-3.2793, -2.0596) (-3.281, -2.0656) (-3.2871, -2.0868) (-3.2961, -2.117) (-3.3057, -2.1469) (-3.3158, -2.1767) (-3.3243, -2.2004) (-3.3276, -2.2093) knots -0.559717 -0.559717 -0.559717 -0.559717 -0.559717 -0.559717 -0.533333 -0.466667 -0.426673 -0.426673 -0.426673 -0.426673 -0.426673 -0.426673
  spline S35 degree 5 poles (-3.3276, -2.2093) (-3.3297, -2.2152) (-3.3373, -2.2359) (-3.3509, -2.2712) (-3.3713, -2.3209) (-3.4, -2.3844) (-3.4356, -2.4558) (-3.474, -2.5265) (-3.5069, -2.5824) (-3.5329, -2.624) (-3.5507, -2.6516) (-3.5598, -2.6654) knots -0.426673 -0.426673 -0.426673 -0.426673 -0.426673 -0.426673 -0.4 -0.333333 -0.266667 -0.2 -0.133333 -0.066667 0 0 0 0 0 0
  arc A28 (-3.5598, -2.6654) -> (-5.9474, -3.5643) centre (-3.3425, -6.8632) ccw
  arc A29 (-5.9474, -3.5643) -> (-5.9442, -3.9339) centre (2.4092, -3.6756) ccw
  arc A30 (-5.9442, -3.9339) -> (-3.5411, -4.7907) centre (-3.3976, -0.5897) ccw
  spline S36 degree 5 poles (-3.5411, -4.7907) (-3.5318, -4.8043) (-3.5135, -4.8316) (-3.4868, -4.8727) (-3.4528, -4.9281) (-3.4132, -4.998) (-3.3764, -5.0688) (-3.3466, -5.1318) (-3.3253, -5.1811) (-3.3111, -5.2162) (-3.3031, -5.2367) (-3.3009, -5.2426) knots 0 0 0 0 0 0 0.066667 0.133333 0.2 0.266667 0.333333 0.4 0.426673 0.426673 0.426673 0.426673 0.426673 0.426673
  spline S37 degree 5 poles (-3.3009, -5.2426) (-3.2975, -5.2514) (-3.2886, -5.275) (-3.2779, -5.3046) (-3.2678, -5.3344) (-3.2582, -5.3644) (-3.2518, -5.3855) (-3.25, -5.3915) knots 0.426673 0.426673 0.426673 0.426673 0.426673 0.426673 0.466667 0.533333 0.559717 0.559717 0.559717 0.559717 0.559717 0.559717
  spline S38 degree 5 poles (-3.25, -5.3915) (-3.2481, -5.3975) (-3.2418, -5.4186) (-3.2331, -5.4489) (-3.2249, -5.4793) (-3.2174, -5.5098) (-3.2117, -5.5344) (-3.2096, -5.5436) knots -0.559717 -0.559717 -0.559717 -0.559717 -0.559717 -0.559717 -0.533333 -0.466667 -0.426673 -0.426673 -0.426673 -0.426673 -0.426673 -0.426673
  spline S39 degree 5 poles (-3.2096, -5.5436) (-3.2082, -5.5497) (-3.2035, -5.5713) (-3.1958, -5.6083) (-3.1861, -5.6611) (-3.1759, -5.7301) (-3.1672, -5.8094) (-3.1613, -5.8895) (-3.1588, -5.9544) (-3.1581, -6.0035) (-3.1582, -6.0363) (-3.1584, -6.0528) knots -0.426673 -0.426673 -0.426673 -0.426673 -0.426673 -0.426673 -0.4 -0.333333 -0.266667 -0.2 -0.133333 -0.066667 0 0 0 0 0 0
  arc A31 (-3.1584, -6.0528) -> (-4.6811, -8.0999) centre (-0.706, -9.4668) ccw
  arc A32 (-4.6811, -8.0999) -> (-4.4785, -8.4091) centre (2.4092, -3.6756) ccw
  arc A33 (-4.4785, -8.4091) -> (-1.9937, -7.8306) centre (-4.1442, -4.2189) ccw
  spline S40 degree 5 poles (-1.9937, -7.8306) (-1.9785, -7.837) (-1.9483, -7.8501) (-1.9036, -7.8703) (-1.8451, -7.8985) (-1.774, -7.9359) (-1.7048, -7.9755) (-1.6456, -8.0125) (-1.6011, -8.0424) (-1.5702, -8.0642) (-1.5523, -8.0772) (-1.5472, -8.0809) knots 0 0 0 0 0 0 0.066667 0.133333 0.2 0.266667 0.333333 0.4 0.426673 0.426673 0.426673 0.426673 0.426673 0.426673
  spline S41 degree 5 poles (-1.5472, -8.0809) (-1.5396, -8.0865) (-1.5194, -8.1015) (-1.4944, -8.1206) (-1.4698, -8.1402) (-1.4455, -8.1603) (-1.4287, -8.1746) (-1.4239, -8.1787) knots 0.426673 0.426673 0.426673 0.426673 0.426673 0.426673 0.466667 0.533333 0.559717 0.559717 0.559717 0.559717 0.559717 0.559717
  spline S42 degree 5 poles (-1.4239, -8.1787) (-1.4192, -8.1827) (-1.4024, -8.197) (-1.3787, -8.2178) (-1.3554, -8.239) (-1.3325, -8.2606) (-1.3145, -8.2781) (-1.3078, -8.2848) knots -0.559717 -0.559717 -0.559717 -0.559717 -0.559717 -0.559717 -0.533333 -0.466667 -0.426673 -0.426673 -0.426673 -0.426673 -0.426673 -0.426673
  spline S43 degree 5 poles (-1.3078, -8.2848) (-1.3033, -8.2892) (-1.2876, -8.3047) (-1.2611, -8.3318) (-1.2245, -8.371) (-1.1786, -8.4234) (-1.1284, -8.4854) (-1.0801, -8.5497) (-1.0429, -8.6029) (-1.0158, -8.6438) (-0.9981, -8.6715) (-0.9894, -8.6855) knots -0.426673 -0.426673 -0.426673 -0.426673 -0.426673 -0.426673 -0.4 -0.333333 -0.266667 -0.2 -0.133333 -0.066667 0 0 0 0 0 0
  circle A34 centre (2.4092, -3.6756) radius 7.6384
  constraint concentric A0 A34
extrude "Extrude4" cut sketch "Sketch5" against normal blind 12.7 contours A1 A2 A3 A34 | A31 A32 A33 A34 | A4 A5 A6 A34 | A28 A29 A30 A34 | A7 A8 A9 A34 | A25 A26 A27 A34 | A10 A11 A12 A34 | A22 A23 A24 A34 | A19 A20 A21 A34 | A13 A14 A15 A34 | A16 A17 A18 A34
fillet "Fillet1" radius 0.508 22 edges at (0.2276, -3.4933, 3.4925) (1.3991, -2.9458, 3.4925) (-2.7853, -3.9535, 3.4925) (-4.0667, -3.7808, 3.4925) (-6.8502, -2.5391, 3.4925) (3.6848, -0.9297, 3.4925) (4.3743, 0.1642, 3.4925) (5.2072, 3.096, 3.4925) (5.1959, 4.3891, 3.4925) (3.6029, 8.3874, 3.4925) (4.3115, 7.3058, 3.4925) (1.282, 10.363, 3.4925) (0.1011, 10.8898, 3.4925) (-2.9194, 11.297, 3.4925) (-4.1977, 11.1017, 3.4925) (-7.9286, 8.9559, 3.4925) (-6.9588, 9.8112, 3.4925) (-9.9071, 5.1336, 3.4925) (-9.5537, 6.3775, 3.4925) (-9.8803, 2.0859, 3.4925) (-9.5051, 0.8485, 3.4925) (-7.8348, -1.7009, 3.4925)
